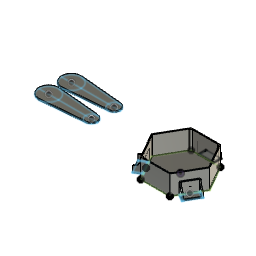
robotic-arm (Autodesk Fusion 360 design; units mm, degrees)
Autodesk Fusion 360 part; units mm, degrees
sketch "Sketch1" plane through (0, 0, 0) normal (0, 0, 1) x (1, 0, 0)
  line L0 (75, 0) -> (37.5, 64.9519)
  line L1 (37.5, 64.9519) -> (-37.5, 64.9519)
  line L2 (-37.5, 64.9519) -> (-75, 0)
  line L3 (-75, 0) -> (-37.5, -64.9519)
  line L4 (-37.5, -64.9519) -> (37.5, -64.9519)
  line L5 (37.5, -64.9519) -> (75, 0)
  line L6 (-20, 84.9519) -> (20, 84.9519)
  line L7 (20, 84.9519) -> (20, 64.9519)
  line L8 (20, 64.9519) -> (-20, 64.9519)
  line L9 (-20, 64.9519) -> (-20, 84.9519)
  line L10 (-20, 84.9519) -> (-17, 84.9519)
  line L11 (-17, 84.9519) -> (-17, 64.9519)
  line L12 (-17, 64.9519) -> (-20, 64.9519)
  line L13 (-20, 64.9519) -> (-20, 84.9519)
  line L14 (20, 84.9519) -> (17, 84.9519)
  line L15 (17, 84.9519) -> (17, 64.9519)
  line L16 (17, 64.9519) -> (20, 64.9519)
  line L17 (20, 64.9519) -> (20, 84.9519)
  line L18 (66.25, -15.1554) -> (64.75, -17.7535)
  line L19 (66.25, -15.1554) -> (83.5705, -25.1554)
  line L20 (65.0705, -57.1984) -> (63.5705, -59.7965)
  line L21 (47.75, -47.1984) -> (65.0705, -57.1984)
  line L22 (83.5705, -25.1554) -> (66.25, -15.1554)
  line L23 (82.0705, -27.7535) -> (83.5705, -25.1554)
  line L24 (64.75, -17.7535) -> (82.0705, -27.7535)
  line L25 (83.5705, -25.1554) -> (63.5705, -59.7965)
  line L26 (46.25, -49.7965) -> (47.75, -47.1984)
  line L27 (46.25, -49.7965) -> (66.25, -15.1554)
  line L28 (63.5705, -59.7965) -> (46.25, -49.7965)
  line L29 (63.5705, -59.7965) -> (46.25, -49.7965)
  line L30 (-46.25, -49.7965) -> (-47.75, -47.1984)
  line L31 (-46.25, -49.7965) -> (-63.5705, -59.7965)
  line L32 (-82.0705, -27.7535) -> (-83.5705, -25.1554)
  line L33 (-64.75, -17.7535) -> (-82.0705, -27.7535)
  line L34 (-63.5705, -59.7965) -> (-46.25, -49.7965)
  line L35 (-65.0705, -57.1984) -> (-63.5705, -59.7965)
  line L36 (-47.75, -47.1984) -> (-65.0705, -57.1984)
  line L37 (-63.5705, -59.7965) -> (-83.5705, -25.1554)
  line L38 (-66.25, -15.1554) -> (-64.75, -17.7535)
  line L39 (-66.25, -15.1554) -> (-46.25, -49.7965)
  line L40 (-83.5705, -25.1554) -> (-66.25, -15.1554)
  line L41 (-83.5705, -25.1554) -> (-66.25, -15.1554)
  line L42 (47.75, -47.1984) -> (50.3481, -48.6984)
  line L43 (50.3481, -48.6984) -> (68.8481, -16.6554)
  line L44 (68.8481, -16.6554) -> (66.25, -15.1554)
  line L45 (66.25, -15.1554) -> (47.75, -47.1984)
  line L46 (-47.75, -47.1984) -> (-50.3481, -48.6984)
  line L47 (-50.3481, -48.6984) -> (-67.3481, -19.2535)
  line L48 (-67.3481, -19.2535) -> (-64.75, -17.7535)
  line L49 (-64.75, -17.7535) -> (-47.75, -47.1984)
  line L50 (17, 64.9519) -> (17, 67.9519)
  line L51 (17, 67.9519) -> (-17, 67.9519)
  line L52 (-17, 67.9519) -> (-17, 64.9519)
  line L53 (-17, 64.9519) -> (17, 64.9519)
  circle A0 centre (37.5, -64.9519) radius 5
  circle A1 centre (-37.5, -64.9519) radius 5
  circle A2 centre (-37.5, 64.9519) radius 5
  circle A3 centre (37.5, 64.9519) radius 5
  line L54 (-367.5273, 61.5103) -> (-217.5273, 61.5103)
  circle A4 centre (-342.5273, 61.5103) radius 25
  circle A5 centre (-232.5273, 61.5103) radius 15
  line L55 (-231.1637, 76.4482) -> (-340.2546, 86.4068)
  line L56 (-231.1637, 46.5724) -> (-340.2546, 36.6138)
  line L57 (-234.4618, 21.3218) -> (-343.5527, 31.2804)
  line L58 (-370.8255, 6.3839) -> (-220.8255, 6.3839)
  circle A6 centre (-235.8255, 6.3839) radius 15
  line L59 (-234.4618, -8.554) -> (-343.5527, -18.5126)
  circle A7 centre (-345.8255, 6.3839) radius 25
  point P0 (56.25, -32.476)
  point P1 (56.25, -32.476)
  point P2 (-56.25, -32.476)
  point P3 (-56.25, -32.476)
  dimension "d1" = 75
  dimension "d5" = 40
  dimension "d6" = 20
  dimension "d7" = 3
  dimension "d8" = 3
  dimension "d9" = 40
  dimension "d10" = 20
  dimension "d11" = 3
  dimension "d12" = 3
  dimension "d13" = 40
  dimension "d14" = 20
  dimension "d15" = 3
  dimension "d16" = 3
  dimension "d31" = 3
  dimension "d32" = 3
  dimension "d42" = 10
  dimension "d43" = 10
  dimension "d44" = 10
  dimension "d45" = 10
  dimension "d48" = 150
  dimension "d49" = 50
  dimension "d50" = 30
  dimension "d51" = 150
  dimension "d52" = 50
  dimension "d53" = 30
  constraint horizontal L6
  constraint vertical L7
  constraint horizontal L8
  constraint vertical L9
  constraint horizontal L10
  constraint vertical L11
  constraint horizontal L12
  constraint vertical L13
  constraint coincident L8 L11.end
  constraint horizontal L14
  constraint vertical L15
  constraint horizontal L16
  constraint vertical L17
  constraint coincident L8 L15.end
  constraint coincident L20.start L25
  constraint coincident L23.start L25
  constraint coincident L32.start L37
  constraint coincident L35.start L37
  constraint midpoint L1 L8
  constraint midpoint L27 P1
  constraint coincident L5 P1
  constraint coincident P1 P0
  constraint midpoint L3 P3
  constraint midpoint L39 P3
  constraint coincident P3 P2
  constraint perpendicular L42 L43
  constraint parallel L42 L44
  constraint parallel L43 L45
  constraint coincident L21 L42.end
  constraint perpendicular L5 L42
  constraint perpendicular L46 L47
  constraint parallel L46 L48
  constraint parallel L47 L49
  constraint perpendicular L3 L46
  constraint perpendicular L50 L51
  constraint parallel L50 L52
  constraint parallel L51 L53
  constraint coincident L15 L50.end
  constraint perpendicular L19 L27
  constraint perpendicular L22 L27
  constraint perpendicular L19 L25
  constraint perpendicular L26 L28
  constraint coincident L4.end L5.start
  constraint coincident L3.end L4.start
  constraint coincident L1.end L2.start
  constraint coincident L0.end L1.start
  constraint horizontal L54
  constraint coincident L54 A4.centre
  constraint coincident L54.start A4
  constraint coincident L54 A5.centre
  constraint coincident L54.end A5
  constraint coincident A5 L55.start
  constraint coincident A4 L55.end
  constraint tangent A4 L55
  constraint coincident A5 L56.start
  constraint coincident A4 L56.end
  constraint tangent A4 L56
  constraint horizontal L58
  constraint coincident A7.centre L58
  constraint coincident L58.start A7
  constraint coincident A6.centre L58
  constraint coincident L58.end A6
  constraint coincident L57.start A6
  constraint coincident L57.end A7
  constraint tangent L57 A7
  constraint coincident L59.start A6
  constraint coincident L59.end A7
  constraint tangent L59 A7
  measures "d1" distance of L0.start origin
  measures "d5" distance of L6.start L6.end
  measures "d6" distance of L6.end L7.end
  measures "d7" distance of L6.start L10.end
  measures "d8" distance of L6.end L14.end
  measures "d9" distance of L26.start L18.start
  measures "d10" distance of L18.start L19.end
  measures "d11" distance of L26.start L21.start
  measures "d12" distance of L18.end L18.start
  measures "d13" distance of L38.start L30.start
  measures "d14" distance of L30.start L31.end
  measures "d15" distance of L38.start L33.start
  measures "d16" distance of L30.end L30.start
  measures "d31" distance of L21.start L42.end
  measures "d32" distance of L15.end L50.end
  measures "d42" diameter of A0
  measures "d43" diameter of A1
  measures "d44" diameter of A2
  measures "d45" diameter of A3
  measures "d48" distance of L54.start L54.end
  measures "d49" diameter of A4
  measures "d50" diameter of A5
  measures "d51" distance of L58.end L58.start
  measures "d52" diameter of A7
  measures "d53" diameter of A6
extrude "Extrude1" add sketch "Sketch1" along normal blind 50 contours L0 L1 L2 L3 L4 L5 L8 L12 L16 L18 L26 L27 L30 L38 L39 L45 L49 L53 A0 A1 A2 A3 | L0 L1 A3 | L4 L5 A0 | L1 L2 A2 | L3 L4 A1 picked at (35.2391, 62.5152) picked at (34.6213, -63.2899) picked at (-34.2593, 64.2122) picked at (-34.2593, -64.2122) makes body 1
shell "Shell1" thickness 2 removed faces 1 at (5.6667, -9.815, 50) on bodies 1
extrude "Extrude2" add sketch "Sketch1" along normal blind 30 separate body contours L5 L18 L19 L22 L24 L27 L43 L44 L45 | L5 L21 L24 L27 L42 L43 L45 | L19 L22 L23 L24 L25 L43 | L1 L6 L7 L8 L14 L15 L16 L17 L50 | L5 L20 L21 L25 L26 L27 L28 L29 L42 | L21 L24 L25 L43 | L1 L8 L11 L15 L50 L51 L52 L53 | L1 L6 L8 L9 L10 L11 L12 L13 L52 | L6 L11 L15 L51 | L3 L30 L31 L34 L35 L36 L37 L39 L46 | L3 L32 L33 L37 L38 L39 L40 L41 L48 | L3 L33 L36 L39 L46 L47 L48 L49 | L33 L36 L37 L47 makes body 2 at (6.6667, 64.9519, 10) makes body 3 at (70.2372, -48.2495, 20) makes body 4 at (-70.2372, -48.2495, 20)
extrude "Extrude3" cut sketch "Sketch1" along normal blind 30 from surface at 3 contours L21 L24 L25 L43 | L6 L11 L15 L51 | L33 L36 L37 L47 bodies 2 3 4
sketch "Sketch2" plane through (10, 17.3205, 0) normal (0.5, 0.866025, 0) x (-0.866025, 0.5, 0)
  line L0 (-84.9519, 0) -> (-64.9519, 0)
  line L1 (-64.9519, 0) -> (-64.9519, 30)
  line L2 (-64.9519, 30) -> (-84.9519, 30)
  line L3 (-84.9519, 30) -> (-84.9519, 0)
  circle A0 centre (-84.9519, 30) radius 15
  dimension "d22" = 30
  constraint coincident L2.end L3.start
  measures "d22" diameter of A0
sketch "Sketch3" plane through (20, 0, 0) normal (1, 0, 0) x (0, 1, 0)
  line L0 (64.9519, 0) -> (84.9519, 0)
  line L1 (84.9519, 0) -> (84.9519, 30)
  line L2 (84.9519, 30) -> (64.9519, 30)
  line L3 (64.9519, 30) -> (64.9519, 0)
  circle A0 centre (84.9519, 30) radius 15
  dimension "d23" = 30
  constraint coincident L1.end L2.start
  measures "d23" diameter of A0
extrude "Extrude4" cut sketch "Sketch3" against normal blind 75 contours L1 L2 A0 picked at (77.8989, 22.9469) bodies 2
extrude "Extrude5" cut sketch "Sketch2" against normal blind 50 contours L2 L3 A0 picked at (-84.2403, 20.0509) bodies 3
sketch "Sketch4" plane through (-10, 17.3205, 0) normal (-0.5, 0.866025, 0) x (-0.866025, -0.5, 0)
  line L0 (64.9519, 0) -> (84.9519, 0)
  line L1 (84.9519, 0) -> (84.9519, 30)
  line L2 (84.9519, 30) -> (64.9519, 30)
  line L3 (64.9519, 30) -> (64.9519, 0)
  circle A0 centre (84.9519, 30) radius 15
  dimension "d28" = 30
  constraint coincident L1.end L2.start
  measures "d28" diameter of A0
extrude "Extrude6" cut sketch "Sketch4" against normal blind 40 contours L1 L2 A0 picked at (84.2403, 20.0509) bodies 4
sketch "Sketch5" plane through (0, 67.9519, 0) normal (0, 1, 0) x (-1, 0, 0)
  line L0 (17, 30) -> (-17, 30)
  line L1 (-17, 30) -> (-17, 3)
  line L2 (-17, 3) -> (17, 3)
  line L3 (17, 3) -> (17, 30)
  circle A0 centre (0, 16.5) radius 1
  dimension "d33" = 2
  measures "d33" diameter of A0
sketch "Sketch6" plane through (58.8481, -33.976, 0) normal (0.866025, -0.5, 0) x (0.5, 0.866025, 0)
  line L0 (17, 30) -> (-17, 30)
  line L1 (-17, 30) -> (-17, 3)
  line L2 (-17, 3) -> (17, 3)
  line L3 (17, 3) -> (17, 30)
  circle A0 centre (-0.0409, 16.5) radius 1
  dimension "d34" = 2
  measures "d34" diameter of A0
sketch "Sketch7" plane through (-58.8481, -33.976, 0) normal (-0.866025, -0.5, 0) x (0.5, -0.866025, 0)
  line L0 (17, 30) -> (-17, 30)
  line L1 (-17, 30) -> (-17, 3)
  line L2 (-17, 3) -> (17, 3)
  line L3 (17, 3) -> (17, 30)
  circle A0 centre (0, 16.5) radius 1
  dimension "d35" = 2
  measures "d35" diameter of A0
extrude "Extrude7" cut sketch "Sketch7" against normal blind 5 contours A0 bodies 1 4
extrude "Extrude8" cut sketch "Sketch5" against normal blind 4 contours A0 bodies 1 2
extrude "Extrude9" cut sketch "Sketch6" against normal blind 6 contours A0 bodies 1 3
extrude "Extrude10" add sketch "Sketch1" along normal blind 50 contours L0 L1 A3 | L4 L5 A0 | L1 L2 A2 | L3 L4 A1 picked at (35.2391, 62.5152) picked at (34.6213, -63.2899) picked at (-34.2593, 64.2122) picked at (-34.2593, -64.2122) bodies 1
extrude "Extrude11" add sketch "Sketch1" along normal blind 3 separate body contours L54 A4 | L54 A4 | L54 A4 A5 L55 | L54 A4 A5 L56 | L54 A5 | L54 A5 | L57 L58 A6 A7 | L58 A6 | L58 A7 | L58 A6 | L58 A6 L59 A7 | L58 A7 makes body 5 at (-307.1891, 1.4046, 3) makes body 6 at (-303.891, 56.531, 0)
